Autodesk Fusion 360 part; units mm, degrees
(part 2 of 2)
extrude "Estrusione19" cut sketch "Schizzo15" against normal up to surface (1.6 mm away) contours L4 A0 L5 A1 L6 L7 L8 L9 | A2 L10 A3 L11 L12 L13 L14 L15 | L24 L25 L26 L27 bodies 3 in component "case"
sketch "Schizzo16" plane through (-16, 0, 0) normal (-1, 0, 0) x (0, -1, 0) in component "case"
  line L0 (-80.2, -0.2) -> (-80.2, 80.2)
  line L1 (-80.2, 80.2) -> (0.2, 80.2)
  line L2 (0.2, 80.2) -> (0.2, -0.2)
  line L3 (0.2, -0.2) -> (-80.2, -0.2)
  line L4 (-81.8, 81.8) -> (-81.8, -1.8)
  line L5 (-81.8, -1.8) -> (1.8, -1.8)
  line L6 (1.8, -1.8) -> (1.8, 81.8)
  line L7 (1.8, 81.8) -> (-81.8, 81.8)
  line L8 (0, 80) -> (0, 0)
  line L9 (0, 0) -> (-80, 0)
  line L10 (-80, 0) -> (-80, 80)
  line L11 (-80, 80) -> (0, 80)
  line L12 (-1.2, 78.8) -> (-1.2, 1.2)
  line L13 (-1.2, 1.2) -> (-78.8, 1.2)
  line L14 (-78.8, 1.2) -> (-78.8, 78.8)
  line L15 (-78.8, 78.8) -> (-1.2, 78.8)
  dimension "d169" = 0.2
  dimension "d170" = 1.4
extrude "Estrusione20" add sketch "Schizzo16" along normal blind 1.2 separate body contours L0 L1 L2 L3 | L4 L5 L6 L7 | L8 L9 L10 L11 | L12 L13 L14 L15 makes body 5 in component "case"
extrude "Estrusione21" add sketch "Schizzo16" against normal blind 3 contours L8 L9 L10 L11 bodies 5 in component "case"
sketch "Schizzo17" plane through (-16, 0, 0) normal (1, 0, 0) x (0, 1, 0) in component "case"
  line L0 (78.8, 78.8) -> (1.2, 78.8)
  line L1 (1.2, 78.8) -> (1.2, 1.2)
  line L2 (1.2, 1.2) -> (78.8, 1.2)
  line L3 (78.8, 1.2) -> (78.8, 78.8)
  circle A0 centre (76.3, 2.7) radius 2.5
  circle A1 centre (76.3, 2.7) radius 3.3
  dimension "d175" = 5
  dimension "d176" = 1.5
  dimension "d177" = 0.8
  constraint tangent L3 A0
  measures "d175" diameter of A0
  measures "d176" distance of L2 A0.centre
extrude "Estrusione22" cut sketch "Schizzo17" against normal through all contours L2 A0 picked at (76.8124, 4.0638) bodies 5 in component "case"
extrude "Estrusione23" add sketch "Schizzo17" along normal up to surface (3 mm away) contours L2 L3 A0 A1 picked at (73.4963, 1.5594) bodies 5 in component "case"
sketch "Schizzo18" plane through (-16, 0, 0) normal (1, 0, 0) x (0, 1, 0) in component "case"
  arc A0 (78.8, 4.8541) -> (73.3606, 1.2) centre (76.3, 2.7) ccw
  line L0 (78.8, 4.8541) -> (78.8, 78.8)
  line L1 (78.8, 78.8) -> (1.2, 78.8)
  line L2 (1.2, 78.8) -> (1.2, 1.2)
  line L3 (1.2, 1.2) -> (73.3606, 1.2)
  line L4 (40, 78.8) -> (40, 1.2) construction
  line L5 (60, 8.5) -> (20, 8.5)
  line L6 (20, 8.5) -> (20, 11.5)
  line L7 (20, 11.5) -> (60, 11.5)
  line L8 (60, 11.5) -> (60, 8.5)
  line L9 (60, 8.5) -> (20, 11.5) construction
  line L10 (20, 8.5) -> (60, 11.5) construction
  circle A1 centre (20, 10) radius 1.5
  circle A2 centre (60, 10) radius 1.5
  line L11 (20, 17.5) -> (60, 17.5)
  line L12 (60, 14.5) -> (20, 17.5) construction
  line L13 (20, 14.5) -> (60, 17.5) construction
  line L14 (20, 14.5) -> (20, 17.5)
  circle A3 centre (60, 16) radius 1.5
  circle A4 centre (20, 16) radius 1.5
  line L15 (60, 14.5) -> (20, 14.5)
  line L16 (60, 17.5) -> (60, 14.5)
  line L17 (20, 23.5) -> (60, 23.5)
  line L18 (60, 20.5) -> (20, 23.5) construction
  line L19 (20, 20.5) -> (60, 23.5) construction
  line L20 (20, 20.5) -> (20, 23.5)
  circle A5 centre (60, 22) radius 1.5
  circle A6 centre (20, 22) radius 1.5
  line L21 (60, 20.5) -> (20, 20.5)
  line L22 (60, 23.5) -> (60, 20.5)
  circle A7 centre (20, 70) radius 1.5
  line L23 (20, 56.5) -> (60, 59.5) construction
  line L24 (20, 62.5) -> (20, 65.5)
  line L25 (20, 56.5) -> (20, 59.5)
  line L26 (20, 68.5) -> (20, 71.5)
  line L27 (20, 65.5) -> (60, 65.5)
  line L28 (60, 68.5) -> (20, 71.5) construction
  line L29 (20, 62.5) -> (60, 65.5) construction
  circle A8 centre (60, 58) radius 1.5
  circle A9 centre (60, 70) radius 1.5
  line L30 (60, 62.5) -> (20, 65.5) construction
  circle A10 centre (60, 64) radius 1.5
  line L31 (60, 71.5) -> (60, 68.5)
  line L32 (60, 65.5) -> (60, 62.5)
  line L33 (60, 59.5) -> (60, 56.5)
  line L34 (60, 62.5) -> (20, 62.5)
  line L35 (20, 71.5) -> (60, 71.5)
  line L36 (20, 59.5) -> (60, 59.5)
  circle A11 centre (20, 64) radius 1.5
  line L37 (60, 56.5) -> (20, 56.5)
  line L38 (60, 56.5) -> (20, 59.5) construction
  line L39 (20, 68.5) -> (60, 71.5) construction
  circle A12 centre (20, 58) radius 1.5
  line L40 (60, 68.5) -> (20, 68.5)
  point P0 (40, 10)
  point P1 (40, 16)
  point P2 (40, 22)
  point P3 (40, 64)
  point P4 (40, 70)
  point P5 (40, 58)
  dimension "d181" = 40
  dimension "d182" = 3
  dimension "d185" = 0
  dimension "d186" = 6
  dimension "d189" = 0
  dimension "d190" = 48
  constraint midpoint L1 L4.start
  constraint coincident L3 L4.end
  constraint perpendicular L3 L4
  constraint horizontal L5
  constraint perpendicular L5 L6
  constraint parallel L5 L7
  constraint parallel L6 L8
  constraint coincident L9 P0
  constraint coincident L10 P0
  constraint coincident L4 P0
  constraint coincident L5.end A1
  constraint tangent L5 A1
  constraint coincident L6.end A1
  constraint coincident L5.start A2
  constraint tangent L5 A2
  constraint coincident L7.end A2
  measures "d181" distance of L6.end L7.end
  measures "d182" distance of L5.end L6.end
extrude "Estrusione24" cut sketch "Schizzo18" against normal through all contours L8 A2 | L5 L7 A1 A2 | L8 A2 | L6 A1 | L6 A1 | L14 A4 | L11 A3 A4 L15 | L14 A4 | A3 L16 | A3 L16 | L20 A6 | L17 A5 A6 L21 | L20 A6 | A5 L22 | A5 L22 | A7 L26 | A7 A9 L35 L40 | A7 L26 | A9 L31 | A9 L31 | L24 A11 | L27 A10 L34 A11 | L24 A11 | A10 L32 | A10 L32 | L25 A12 | A8 L36 L37 A12 | L25 A12 | A8 L33 | A8 L33 bodies 5 in component "case"
component "case" placed x (1, 0, 0) y (0, 1, 0) z (0, 0, 1) at (0, 0, 0)
component "elettronica" placed x (1, 0, 0) y (0, 1, 0) z (0, 0, 1) at (0, 0, 0)
equation "d52 = d51"
equation "d54 = d53"
named bodies: "led matrix", "mini d1", "schermo", "telaio", "fondo"
